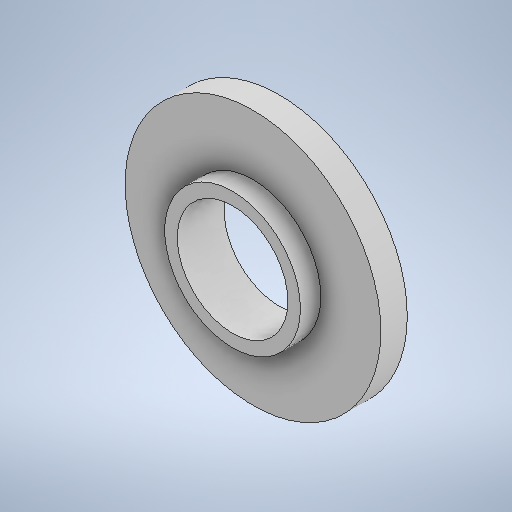
# Autodesk Inventor part: Lower_bushings
Saved by Autodesk Inventor 2025.1 (Build 291241000, 241)
## iProperties
Created: 2025-05-20
Part Number: Lower_bushings
Material: Generic
Document SubType Name: Modeling
Designer: Andreas' PC
Density: 1 g/cm^3
Appearance: Default
Author: Andreas' PC
## iProperties of the stored document Lower_bushings_3DPrint.ipt
Created: 2025-05-27
Part Number: Lower_bushings_3DPrint
Material: Generic
Document SubType Name: Modeling
Designer: Andreas' PC
Density: 1 g/cm^3
Appearance: Default
Author: Andreas' PC
Autodesk Inventor part; units mm, degrees
ref_plane "YZ Plane" through (0, 0, 0) normal (1, 0, 0) x (0, 1, 0)
ref_plane "XZ Plane" through (0, 0, 0) normal (0, 1, 0) x (-1, 0, 0)
ref_plane "XY Plane" through (0, 0, 0) normal (0, 0, 1) x (1, 0, 0)
sketch "Sketch1" plane through (0, 0, 0) normal (0, 0, 1) x (1, 0, 0)
  circle A0 centre (0, 0) radius 8.15
  circle A1 centre (0, 0) radius 10
  circle A2 centre (0, 0) radius 18.85
  dimension "d0" = 16.3
  dimension "d1" = 20
  dimension "d2" = 37.7
  constraints: 3 centre point, 3 coincident
  measures "d0" diameter of A0
  measures "d1" diameter of A1
  measures "d2" diameter of A2
extrude "Extrusion1" add sketch "Sketch1" along normal blind 6.9 contours A1
extrude "Extrusion2" add sketch "Sketch1" along normal blind 3.9 contours A2
equation "\"d0\" = shaft_d"
equation "\"d1\" = i_d"
equation "\"d2\" = o_d"
equation "\"d5\" = spacing"
equation "\"shaft_d\" = 16.3"
equation "\"o_d\" = 37.7"
equation "\"spacing\" = 3.9"
equation "\"i_d\" = 20"
body "Solid1"
